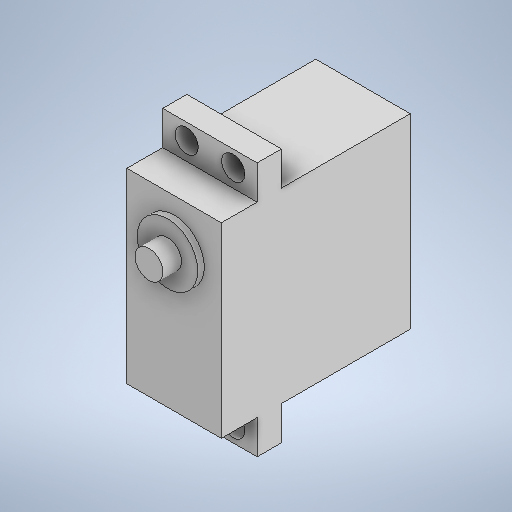
# Autodesk Inventor part: stepper_new
Saved by Autodesk Inventor 2025.1 (Build 291241000, 241)
## iProperties
Created: 2024-11-14
Part Number: stepper_new
Material: Generisch
Document SubType Name: Modeling
Designer: ZOMBULLI
Density: 1 g/cm^3
Appearance: Vorgabe
Author: ZOMBULLI
Autodesk Inventor part; units mm, degrees
ref_plane "YZ Plane" through (0, 0, 0) normal (1, 0, 0) x (0, 1, 0)
ref_plane "XZ Plane" through (0, 0, 0) normal (0, 1, 0) x (-1, 0, 0)
ref_plane "XY Plane" through (0, 0, 0) normal (0, 0, 1) x (1, 0, 0)
sketch "Skizze1" plane through (0, 0, 0) normal (0, 1, 0) x (-1, 0, 0)
  line L0 (10.15, 20.05) -> (-10.15, 20.05)
  line L1 (-10.15, 20.05) -> (-10.15, -20.05)
  line L2 (-10.15, -20.05) -> (10.15, -20.05)
  line L3 (10.15, -20.05) -> (10.15, 20.05)
  line L4 (14.21, 0) -> (-14.21, 0) projected
  line L5 (0, -28.07) -> (0, 28.07) projected
  point P0 (0, 0)
  dimension "d0" = 40.1
  dimension "d1" = 20.3
  constraints: 8 end point, 2 parallel, 1 horizontal, 1 perpendicular, 2 other
  measures "d0" distance of L2.end L0.start
  measures "d1" distance of L1.end L2.end
extrude "Extrusion1" add sketch "Skizze1" along normal blind 40.6
sketch "Skizze2" plane through (0, 0, 0) normal (0, -1, 0) x (1, 0, 0)
  circle A0 centre (0, 9.95) radius 6.5
  line L0 (10.15, -20.05) -> (-10.15, -20.05) projected
  line L1 (0, 28.07) -> (0, -28.07) projected
  point P0 (0, 0)
  dimension "d4" = 13
  dimension "d5" = 30
  dimension "d6" = 0
  constraints: 1 centre point
  measures "d4" diameter of A0
  measures "d5" distance from line of L0 A0.centre
  measures "d6" distance from line of L1 A0.centre
extrude "Extrusion2" add sketch "Skizze2" along normal blind 1.4
sketch "Skizze3" plane through (0, -1.4, 9.95) normal (0, -1, 0) x (1, 0, 0)
  circle A0 centre (0, 0) radius 3
  point P0 (0, -9.95)
  dimension "d9" = 6
  constraints: 1 centre point
  measures "d9" diameter of A0
extrude "Extrusion3" add sketch "Skizze3" along normal blind 4
sketch "Skizze4" plane through (-10.15, 0, 20.05) normal (0, 0, 1) x (1, 0, 0)
  line L0 (20.3, 7.7) -> (0, 7.7)
  line L1 (0, 7.7) -> (0, 12.9)
  line L2 (0, 12.9) -> (20.3, 12.9)
  line L3 (20.3, 12.9) -> (20.3, 7.7)
  line L4 (0, 0) -> (20.3, 0) projected
  line L5 (20.3, 0) -> (20.3, 40.6) projected
  point P0 (10.15, 0)
  point P1 (20.3, 10.3)
  dimension "d12" = 0
  dimension "d13" = 7.7
  dimension "d14" = 5.2
  constraints: 8 end point, 3 parallel, 1 horizontal, 1 midpoint, 1 perpendicular
  measures "d12" distance from line of L5 point (20.3, 10.3)
  measures "d13" distance between parallel lines of L4 L0
  measures "d14" distance of L0.end L1.end
extrude "Extrusion4" add sketch "Skizze4" along normal blind 7.3
sketch "Skizze5" plane through (10.15, 0, -20.05) normal (0, 0, -1) x (-1, 0, 0)
  line L0 (20.3, 7.7) -> (0, 7.7)
  line L1 (0, 7.7) -> (0, 12.9)
  line L2 (0, 12.9) -> (20.3, 12.9)
  line L3 (20.3, 12.9) -> (20.3, 7.7)
  line L4 (0, 0) -> (20.3, 0) projected
  line L5 (20.3, 0) -> (20.3, 40.6) projected
  point P0 (10.15, 0)
  dimension "d17" = 0
  dimension "d20" = 7.7
  dimension "d21" = 5.2
  constraints: 8 end point, 3 parallel, 1 horizontal, 1 perpendicular
  measures "d17" distance between parallel lines of L5 L3
  measures "d20" distance between parallel lines of L0 L4
  measures "d21" distance of L0.end L1.end
extrude "Extrusion5" add sketch "Skizze5" along normal blind 7.3
sketch "Skizze6" plane through (-10.15, 7.7, 20.05) normal (0, -1, 0) x (1, 0, 0)
  circle A0 centre (15.15, 3.85) radius 2.5
  circle A1 centre (5.15, 3.85) radius 2.5
  circle A2 centre (15.15, -43.95) radius 2.5
  circle A3 centre (5.15, -43.95) radius 2.5
  line L0 (10.15, -58.34) -> (10.15, 18.24) projected
  line L1 (0, 7.3) -> (20.3, 7.3) projected
  line L2 (0, 0) -> (20.3, 0) projected
  line L3 (20.3, -40.1) -> (0, -40.1) projected
  point P0 (10.15, -20.05)
  dimension "d22" = 5
  dimension "d23" = 10
  dimension "d29" = 47.8
  dimension "d30" = 3.45
  constraints: 4 centre point, 3 equal radius, 2 horizontal alignment, 2 vertical alignment, 1 other
  measures "d22" diameter of A0
  measures "d23" distance of A1.centre A0.centre
  measures "d29" distance of A2.centre A0.centre
  measures "d30" distance from line of L1 A0.centre
extrude "Extrusion6" cut sketch "Skizze6" against normal blind 7.3
